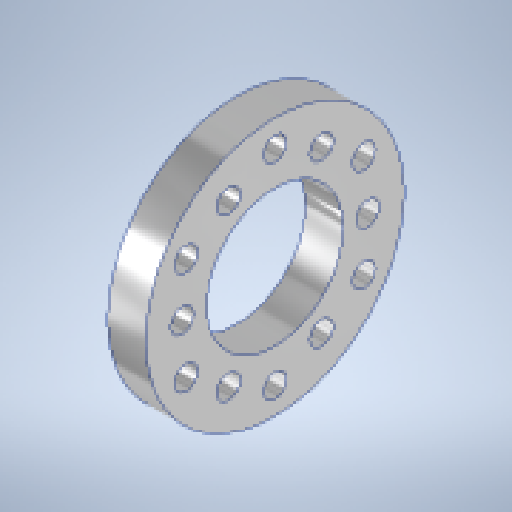
# Autodesk Inventor part: link2part6
Saved by Autodesk Inventor 2024 (Build 280153000, 153)
## iProperties
Created: 2025-02-11
Part Number: link2part6
Material: アルミニウム 6061
Document SubType Name: Modeling
Designer: tanoue_kota
Density: 2.7 g/cm^3
Appearance: アルミニウム - フラット
Mass: 2.28171 g
Surface Area: 22.2282 cm^2
Volume: 2.28171 cm^3
Author: tanoue_kota
Autodesk Inventor part; units mm, degrees
ref_plane "YZ Plane" through (0, 0, 0) normal (1, 0, 0) x (0, 1, 0)
ref_plane "XZ Plane" through (0, 0, 0) normal (0, 1, 0) x (-1, 0, 0)
ref_plane "XY Plane" through (0, 0, 0) normal (0, 0, 1) x (1, 0, 0)
sketch "スケッチ1" plane through (0, 0, 0) normal (1, 0, 0) x (0, 1, 0)
  circle A0 centre (0, 0) radius 17
  dimension "d0" = 34
  constraints: 1 centre point, 1 coincident
  measures "d0" diameter of A0
extrude "押し出し1" add sketch "スケッチ1" along normal blind 5
sketch "スケッチ2" plane through (5, 0, 0) normal (1, 0, 0) x (0, 0, -1)
  circle A0 centre (0, 0) radius 13.5
  circle A1 centre (0, 0) radius 12.23
  line L0 (0, 0) -> (0, 13.5)
  line L1 (0, 0) -> (6.115, 10.5915)
  point P0 (-11.6913, 6.75)
  point P1 (-11.6913, -6.75)
  point P2 (0, -13.5)
  point P3 (11.6913, -6.75)
  point P4 (11.6913, 6.75)
  point P5 (-6.115, 10.5915)
  point P6 (-12.23, 0)
  point P7 (-6.115, -10.5915)
  point P8 (6.115, -10.5915)
  point P9 (12.23, 0)
  dimension "d3" = 27
  dimension "d4" = 24.46
  dimension "d5" = 30
  dimension "d8" = 360
  dimension "d12" = 360
  constraints: 4 coincident, 4 end point, 1 vertical, 1 vertical alignment, 19 other
  measures "d5" angle of L0 L1
hole "穴1" at (5, 13.5, 0) at (5, 6.75, 11.6913) at (5, -6.75, 11.6913) at (5, -13.5, 0) at (5, -6.75, -11.6913) at (5, 6.75, -11.6913) at (5, 10.5915, -6.115) at (5, 10.5915, 6.115) at (5, 0, 12.23) at (5, -10.5915, 6.115) at (5, 0, -12.23) at (5, -10.5915, -6.115) direction (-1, 0, 0) diameter 3.1 end through all
sketch "スケッチ3" plane through (5, 0, 0) normal (1, 0, 0) x (0, 0, -1)
  circle A0 centre (0, 0) radius 9
  dimension "d21" = 18
  constraints: 1 centre point, 1 coincident
  measures "d21" diameter of A0
extrude "押し出し2" cut sketch "スケッチ3" against normal blind 5
